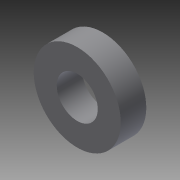
# Autodesk Inventor part: 1.06250.311-rod_part0
Saved by Autodesk Inventor 2014 SP2 (Build 180246200, 246)
## iProperties
Created: 2020-02-04
Part Number: 1.06250.311-rod_part0
Material: Generic
Catalog Web Link: www.cadenas.de
Description: FO1-Rod Part-Bimba FLAT-1
Vendor: BIMBA
Document SubType Name: Modeling
Designer: psadmin
Manufacturer: BIMBA
Mass: 3.51373 g
Surface Area: 18.7422 cm^2
Volume: 3.51373 cm^3
Density: 1 g/cm^3
Appearance: PSOLRGB-180-180-180
Category: PARTsolutions
Company: BIMBA
Title: 1.06250.311-rod_part0
Author: Cadenas PARTsolutions
Comments: Bimba FLAT-1
PSOL_IDENT_0: {$CADENAS_DATA\23d-libs\bimba\bimba_brand\bimba_imperial\bimba_full_line\flat_cylinders\fo1\fo1_rod_
PSOL_IDENT_1: part.prj},198 {VTYP=3D},{NB=1.06250.311-rod_part0},{LINA=1.06250.311-rod_part0},{NN=FO1-Rod Part},{D
PSOL_IDENT_2: ATE=22.01.2020 09:06:03},{GEOMDATE=02.05.2017 08:19:00},{VERSION=},{LINEID=30},{WBVAR=L,BCD},{WBNUME
PSOL_IDENT_3: RIC=L,BCD}  {NB=1.06250.311-rod_part0},{LINA=1.06250.311-rod_part0},{KT=DUMMY},{PN=1.06250.311-rod_p
PSOL_IDENT_4: art0},{BORE=1.06250000},{L=0.311},{TDIN=1.06200000},{F=0.50000000},{BCD=0},{A=2.000}
NN: FO1-Rod Part
NT: Bimba FLAT-1
NB: 1.06250.311-rod_part0
NBSYN: $PN.
LINA: 1.06250.311-rod_part0
PN: 1.06250.311-rod_part0
BORE: 1.0625
L: 0.311
TDIN: 1.062
F: 0.5
BCD: 0
A: 2
SUPPLIER: BIMBA
ARTICLENO: 1.06250.311-rod_part0
BOMINFO: 1.06250.311-rod_part0
CREATOR: CADENAS GmbH
Autodesk Inventor part; units mm, degrees
ref_plane "YZ Plane" through (0, 0, 0) normal (1, 0, 0) x (0, 1, 0)
ref_plane "XZ Plane" through (0, 0, 0) normal (0, 1, 0) x (-1, 0, 0)
ref_plane "XY Plane" through (0, 0, 0) normal (0, 0, 1) x (1, 0, 0)
sketch "Sketch_1" plane through (0, 0, 0) normal (1, 0, 0) x (0, 1, 0)
  line L0 (0, -7.8994) -> (0, 0)
  line L1 (6.35, 0) -> (6.35, -7.8994)
  line L2 (6.35, -7.8994) -> (13.4874, -7.8994)
  line L3 (13.4874, -7.8994) -> (13.4874, 0)
  line L4 (13.4874, 0) -> (6.35, 0)
  constraints: 10 end point
revolve "Revolution1" add sketch "Sketch_1" angle 360 about axis through (0, 0, -7.8994) along (0, 0, -1)
ref_plane "part_to_rod_XY" through (0, 0, -3.9497) normal (0, 0, 1) x (1, 0, 0)
ref_plane "part_to_rod_YZ" through (0, 0, -3.9497) normal (1, 0, 0) x (0, 1, 0)
ref_plane "part_to_rod_ZX" through (0, 0, -3.9497) normal (0, 1, 0) x (0, 0, 1)
body "Solid1"
